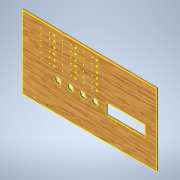
# Autodesk Inventor part: wooden-panel
Saved by Autodesk Inventor 2021 (Build 250183000, 183)
## iProperties
Created: 2020-05-18
Part Number: wooden-panel
Material: Laminated Veneer Lumber
Document SubType Name: Modeling
Designer: Johansson
Density: 0.51 g/cm^3
Appearance: Plywood - New
Author: Johansson
Autodesk Inventor part; units mm, degrees
ref_plane "YZ Plane" through (0, 0, 0) normal (1, 0, 0) x (0, 1, 0)
ref_plane "XZ Plane" through (0, 0, 0) normal (0, 1, 0) x (-1, 0, 0)
ref_plane "XY Plane" through (0, 0, 0) normal (0, 0, 1) x (1, 0, 0)
sketch "Sketch1" plane through (0, 0, 0) normal (0, 0, 1) x (1, 0, 0)
  line L0 (0, 0) -> (630, 0)
  line L1 (630, 0) -> (630, 260)
  line L2 (630, 260) -> (0, 267)
  line L3 (0, 267) -> (0, 0)
  dimension "d0" = 630
  dimension "d1" = 260
  dimension "d2" = 267
  constraints: 8 end point, 1 horizontal, 1 parallel, 1 perpendicular
  measures "d0" distance of L0.start L0.end
  measures "d1" distance of L0.end L1.end
  measures "d2" distance of L2.end L0.start
extrude "Extrusion1" add sketch "Sketch1" along normal blind 8
sketch "Sketch2" plane through (0, 0, 8) normal (0, 0, 1) x (1, 0, 0)
  line L0 (394, 88.3333) -> (577, 88.3333)
  line L1 (577, 88.3333) -> (577, 35.3333)
  line L2 (577, 35.3333) -> (394, 35.3333)
  line L3 (394, 35.3333) -> (394, 88.3333)
  line L4 (630, 0) -> (630, 260) projected
  line L5 (0, 0) -> (630, 0) projected
  dimension "d5" = 183
  dimension "d6" = 53
  dimension "d7" = 53
  dimension "d8" = 35.3333
  constraints: 8 end point, 2 parallel, 1 horizontal, 1 perpendicular
  measures "d5" distance of L1.end L2.end
  measures "d6" distance of L0.end L1.end
  measures "d7" distance between parallel lines of L1 L4
  measures "d8" distance between parallel lines of L5 L2
extrude "Extrusion2" cut sketch "Sketch2" against normal up to next
sketch "Sketch3" plane through (0, 0, 8) normal (0, 0, 1) x (1, 0, 0)
  circle A0 centre (150, 113.3333) radius 4
  line L0 (150, 314.3416) -> (150, 72.5342) construction
  line L1 (577, 88.3333) -> (577, 35.3333) projected
  line L2 (394, 88.3333) -> (577, 88.3333) projected
  line L3 (0, 267) -> (0, 0) projected
  circle A1 centre (130, 113.3333) radius 0.5
  line L4 (150, 113.3333) -> (107.4408, 113.3333) construction
  circle A2 centre (90, 113.3333) radius 0.5
  dimension "d11" = 8
  dimension "d13" = 25
  dimension "d36" = 150
  dimension "d45" = 20
  dimension "d46" = 1
  dimension "d47" = 40
  constraints: 4 end point, 3 centre point, 3 point on line, 1 equal radius, 1 horizontal, 1 vertical
  measures "d11" diameter of A0
  measures "d13" distance from line of L2 L4.start
  measures "d36" distance between parallel lines of L3 L0
  measures "d45" distance of L4.start A1.centre
  measures "d46" diameter of A1
  measures "d47" distance of A1.centre A2.centre
extrude "Extrusion3" cut sketch "Sketch3" against normal up to next
sketch "Sketch5" plane through (0, 0, 8) normal (0, 0, 1) x (1, 0, 0)
  line L0 (539.6603, 61.8333) -> (142.3397, 61.8333) construction
  line L1 (202.9181, 88.3333) -> (312.9941, 88.3333) construction
  line L2 (316.7898, 35.3333) -> (243.2477, 35.3333) construction
  line L3 (577, 35.3333) -> (394, 35.3333) projected
  line L4 (394, 88.3333) -> (577, 88.3333) projected
  circle A0 centre (341, 61.8333) radius 14.5
  line L5 (394, 35.3333) -> (394, 88.3333) projected
  point P0 (0, 0)
  dimension "d26" = 29
  dimension "d27" = 53
  constraints: 6 end point, 3 horizontal, 2 collinear, 2 midpoint, 1 centre point, 1 other
  measures "d26" diameter of A0
  measures "d27" distance from line of A0.centre L5
extrude "Extrusion5" cut sketch "Sketch5" against normal up to next
pattern_linear "Rectangular Pattern3" count 4 spacing 58 along (-1, 0, 0) of "Extrusion5"
pattern_linear "Rectangular Pattern4" count 3 spacing 100 along (1, 0, 0) count 6 spacing 25 along (0, 1, 0) of "Extrusion3"
thicken "Thicken1" operation add thickness 75 both sides no extend neighbours yes toward (0, -1, 0) faces at (210, 0, 2.6667)
sketch "Sketch6" plane through (0, 0, 8) normal (0, 0, 1) x (1, 0, 0)
  circle A0 centre (330, 238.3333) radius 0.5 projected
  circle A1 centre (290, 238.3333) radius 0.5 projected
  circle A2 centre (350, 238.3333) radius 4 projected
  circle A3 centre (230, 238.3333) radius 0.5 projected
  circle A4 centre (190, 238.3333) radius 0.5 projected
  circle A5 centre (250, 238.3333) radius 4 projected
  circle A6 centre (130, 238.3333) radius 0.5 projected
  circle A7 centre (90, 238.3333) radius 0.5 projected
  circle A8 centre (150, 238.3333) radius 4 projected
  circle A9 centre (330, 213.3333) radius 0.5 projected
  circle A10 centre (290, 213.3333) radius 0.5 projected
  circle A11 centre (350, 213.3333) radius 4 projected
  circle A12 centre (230, 213.3333) radius 0.5 projected
  circle A13 centre (190, 213.3333) radius 0.5 projected
  circle A14 centre (250, 213.3333) radius 4 projected
  circle A15 centre (130, 213.3333) radius 0.5 projected
  circle A16 centre (90, 213.3333) radius 0.5 projected
  circle A17 centre (150, 213.3333) radius 4 projected
  circle A18 centre (330, 188.3333) radius 0.5 projected
  circle A19 centre (290, 188.3333) radius 0.5 projected
  circle A20 centre (350, 188.3333) radius 4 projected
  circle A21 centre (230, 188.3333) radius 0.5 projected
  circle A22 centre (190, 188.3333) radius 0.5 projected
  circle A23 centre (250, 188.3333) radius 4 projected
  circle A24 centre (130, 188.3333) radius 0.5 projected
  circle A25 centre (90, 188.3333) radius 0.5 projected
  circle A26 centre (150, 188.3333) radius 4 projected
  circle A27 centre (330, 163.3333) radius 0.5 projected
  circle A28 centre (290, 163.3333) radius 0.5 projected
  circle A29 centre (350, 163.3333) radius 4 projected
  circle A30 centre (230, 163.3333) radius 0.5 projected
  circle A31 centre (190, 163.3333) radius 0.5 projected
  circle A32 centre (250, 163.3333) radius 4 projected
  circle A33 centre (130, 163.3333) radius 0.5 projected
  circle A34 centre (90, 163.3333) radius 0.5 projected
  circle A35 centre (150, 163.3333) radius 4 projected
  circle A36 centre (330, 138.3333) radius 0.5 projected
  circle A37 centre (290, 138.3333) radius 0.5 projected
  circle A38 centre (350, 138.3333) radius 4 projected
  circle A39 centre (230, 138.3333) radius 0.5 projected
  circle A40 centre (190, 138.3333) radius 0.5 projected
  circle A41 centre (250, 138.3333) radius 4 projected
  circle A42 centre (130, 138.3333) radius 0.5 projected
  circle A43 centre (90, 138.3333) radius 0.5 projected
  circle A44 centre (150, 138.3333) radius 4 projected
  circle A45 centre (330, 113.3333) radius 0.5 projected
  circle A46 centre (290, 113.3333) radius 0.5 projected
  circle A47 centre (350, 113.3333) radius 4 projected
  circle A48 centre (230, 113.3333) radius 0.5 projected
  circle A49 centre (190, 113.3333) radius 0.5 projected
  circle A50 centre (250, 113.3333) radius 4 projected
  circle A51 centre (167, 61.8333) radius 14.5 projected
  circle A52 centre (225, 61.8333) radius 14.5 projected
  circle A53 centre (283, 61.8333) radius 14.5 projected
  circle A54 centre (341, 61.8333) radius 14.5 projected
  circle A55 centre (130, 113.3333) radius 0.5 projected
  circle A56 centre (150, 113.3333) radius 4 projected
  circle A57 centre (90, 113.3333) radius 0.5 projected
  line L0 (394, 35.3333) -> (394, 88.3333) projected
  line L1 (394, 88.3333) -> (577, 88.3333) projected
  line L2 (577, 88.3333) -> (577, 35.3333) projected
  line L3 (577, 35.3333) -> (394, 35.3333) projected
  line L4 (0, -75) -> (630, -75) projected
  line L5 (630, -75) -> (630, 260) projected
  line L6 (630, 260) -> (0, 267) projected
  line L7 (0, 267) -> (0, -75) projected
  point P0 (0, 0)
equation "\"d0\" = l_panel"
equation "\"d1\" = wr_panel"
equation "\"d2\" = wl_panel"
equation "\"d3\" = t_panel"
equation "\"d5\" = l_stereo"
equation "\"d6\" = w_stereo"
equation "\"d7\" = d6"
equation "\"d8\" = 0.666667 * d7"
equation "\"d9\" = t_panel"
equation "\"d11\" = r_button"
equation "\"d13\" = l_buttontobutton"
equation "\"d36\" = 3 * l_label"
equation "\"d26\" = r_usboutlet"
equation "\"d27\" = w_stereo"
equation "\"d28\" = t_panel"
equation "\"d32\" = 2 * r_usboutlet"
equation "\"d43\" = w_hidden_panel"
equation "\"d44\" = w_hidden_panel"
equation "\"d39\" = l_label + 2 * l_buttontobutton"
equation "\"d42\" = l_buttontobutton"
equation "\"l_panel\" = 630"
equation "\"wl_panel\" = 267"
equation "\"wr_panel\" = 260"
equation "\"t_panel\" = 8"
equation "\"r_button\" = 8"
equation "\"l_stereo\" = 183"
equation "\"d_stereo\" = 177"
equation "\"w_stereo\" = 53"
equation "\"w_label\" = 15"
equation "\"ro_labelscrew\" = 5"
equation "\"r_labelscrew\" = 2.5"
equation "\"l_buttontobutton\" = 25"
equation "\"r_usboutlet\" = 29"
equation "\"l_fastener_button\" = 19"
equation "\"w_hidden_panel\" = 75"
equation "\"l_label\" = 50"
body "Solid1"
